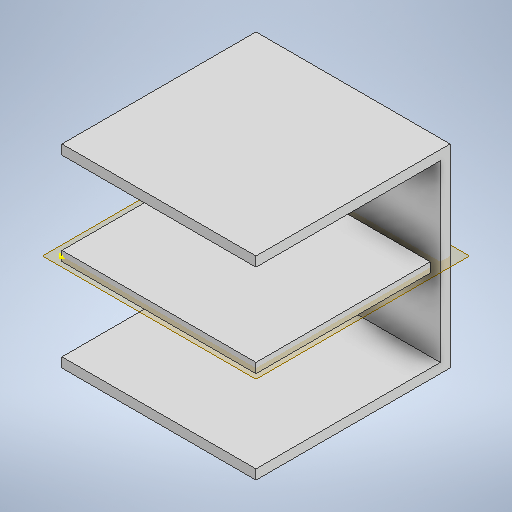
# Autodesk Inventor part: Holstrer
Saved by Autodesk Inventor 2025.3 (Build 293356030, 356C)
## iProperties
Created: 2026-06-23
Part Number: Holstrer
Material: Generic
Document SubType Name: Modeling
Designer: user
Density: 1 g/cm^3
Appearance: Default
Author: user
Autodesk Inventor part; units mm, degrees
ref_plane "YZ Plane" through (0, 0, 0) normal (1, 0, 0) x (0, 1, 0)
ref_plane "XZ Plane" through (0, 0, 0) normal (0, 1, 0) x (-1, 0, 0)
ref_plane "XY Plane" through (0, 0, 0) normal (0, 0, 1) x (1, 0, 0)
sketch "Sketch1" plane through (0, 0, 0) normal (0, 1, 0) x (-1, 0, 0)
  line L0 (0, 0) -> (-200, 0)
  line L1 (-200, 0) -> (-200, -200)
  line L2 (-200, -200) -> (0, -200)
  line L3 (0, -200) -> (0, 0)
  dimension "d0" = 200
  dimension "d1" = 200
  constraints: 8 end point, 2 parallel, 1 horizontal, 1 perpendicular
  measures "d0" distance of L2.end L1.end
  measures "d1" distance of L1.end L0.end
extrude "Extrusion1" add sketch "Sketch1" along normal blind 200
shell "Shell1" thickness 10 removed faces 3 at (66.6667, 66.6667, 0) at (0, 66.6667, -133.3333) at (200, 66.6667, -66.6667)
ref_plane "Work Plane1" through (0, 100, -190) normal (0, 1, 0) x (1, 0, 0)
sketch "Sketch2" plane through (0, 100, -190) normal (0, 1, 0) x (1, 0, 0)
  point P0 (0, -190)
sketch "Sketch3" plane through (0, 100, -190) normal (0, 1, 0) x (1, 0, 0)
  line L0 (0, -190) -> (200, -190)
  line L1 (200, -190) -> (200, -10.3794)
  line L2 (200, -10.3794) -> (0, -10.3794)
  line L3 (0, -10.3794) -> (0, -190)
  constraints: 8 end point, 2 parallel, 1 horizontal, 1 perpendicular
extrude "Extrusion2" add sketch "Sketch3" along normal mid plane 10
body "Solid1"
